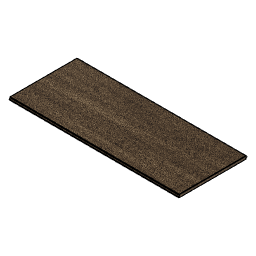
Leaf_Mid (Autodesk Fusion 360 design; units mm, degrees)
Autodesk Fusion 360 part; units mm, degrees
sketch "Sketch1" plane through (0, 0, 0) normal (0, 0, 1) x (1, 0, 0)
  line L0 (-520.7, 210.185) -> (520.7, 210.185)
  line L1 (520.7, 210.185) -> (520.7, -210.185)
  line L2 (520.7, -210.185) -> (-520.7, -210.185)
  line L3 (-520.7, -210.185) -> (-520.7, 210.185)
  line L4 (-520.7, 210.185) -> (520.7, -210.185) construction
  line L5 (520.7, 210.185) -> (-520.7, -210.185) construction
  dimension "d1" = 420.37
  dimension "d2" = 1041.4
  constraint horizontal L0
  constraint perpendicular L0 L1
  constraint parallel L0 L2
  constraint parallel L1 L3
  constraint coincident L4 origin
  constraint coincident L5 origin
  measures "d1" distance of L0.end L1.end
  measures "d2" distance of L0.start L0.end
extrude "Extrude1" add sketch "Sketch1" along normal blind 19.05
sketch "Sketch3" plane through (520.7, 0, 0) normal (1, 0, 0) x (0, 1, 0)
  line L0 (-210.185, 0) -> (210.185, 0)
  line L1 (210.185, 0) -> (210.185, 19.05)
  line L2 (210.185, 19.05) -> (-210.185, 19.05)
  line L3 (-210.185, 19.05) -> (-210.185, 0)
  line L4 (206.375, 0) -> (206.375, 3.175)
  line L5 (206.375, 15.875) -> (206.375, 19.05)
  line L6 (206.375, 3.175) -> (202.565, 4.1959)
  line L7 (202.565, 4.1959) -> (202.565, 8.5041)
  line L8 (202.565, 8.5041) -> (206.375, 9.525)
  line L9 (210.185, 10.5459) -> (210.185, 14.8541) construction
  line L10 (210.185, 14.8541) -> (206.375, 15.875)
  line L11 (206.375, 9.525) -> (210.185, 10.5459)
  line L12 (206.375, 0) -> (210.185, 0)
  line L13 (206.375, 19.05) -> (210.185, 19.05)
  line L14 (210.185, 19.05) -> (210.185, 14.8541)
  line L15 (210.185, 0) -> (210.185, 10.5459)
  line L16 (-202.565, 14.8541) -> (-202.565, 10.5459)
  line L17 (-210.185, 0) -> (-210.185, 4.1959)
  line L18 (-206.375, 19.05) -> (-206.375, 15.875)
  line L19 (-206.375, 9.525) -> (-210.185, 8.5041)
  line L20 (-206.375, 3.175) -> (-206.375, 0)
  line L21 (-206.375, 15.875) -> (-202.565, 14.8541)
  line L22 (-206.375, 19.05) -> (-210.185, 19.05)
  line L23 (-206.375, 0) -> (-210.185, 0)
  line L24 (-210.185, 4.1959) -> (-206.375, 3.175)
  line L25 (-210.185, 19.05) -> (-210.185, 8.5041)
  line L26 (-202.565, 10.5459) -> (-206.375, 9.525)
  line L27 (-210.185, 8.5041) -> (-210.185, 4.1959) construction
  point P0 (210.185, 0)
  dimension "d25" = 105
  dimension "d27" = 19.05
  dimension "d29" = 6.35
  dimension "d30" = 6.35
  dimension "d31" = 3.81
  dimension "d32" = 3.81
  dimension "d33" = 3.81
  dimension "d36" = 105
  dimension "d37" = 19.05
  dimension "d38" = 6.35
  dimension "d39" = 6.35
  dimension "d40" = 3.81
  dimension "d41" = 3.81
  dimension "d42" = 3.81
  constraint vertical L4
  constraint vertical L5
  constraint equal L6 L10
  constraint parallel L6 L10
  constraint equal L4 L5
  constraint equal L7 L9
  constraint equal L8 L11
  constraint equal L6 L8
  constraint perpendicular L9 L12
  constraint perpendicular L5 L13
  constraint perpendicular L13 L14
  constraint perpendicular L12 L15
  constraint equal L21 L24
  constraint parallel L21 L24
  constraint equal L18 L20
  constraint equal L16 L27
  constraint equal L19 L26
  constraint equal L21 L26
  constraint perpendicular L22 L27
  constraint perpendicular L20 L23
  constraint perpendicular L17 L23
  constraint perpendicular L22 L25
  measures "d25" angle of L6 L7
  measures "d27" distance of L4.start L5.end
  measures "d29" distance of L5.start L8.end
  measures "d30" distance of L4.end L8.end
  measures "d31" distance of L7 L8.end
  measures "d32" distance of L9 L8.end
  measures "d33" distance of L4.start P0
  measures "d36" angle of L16 L21
  measures "d37" distance of L20.end L18.start
  measures "d38" distance of L20.start L19.start
  measures "d39" distance of L18.end L19.start
  measures "d40" distance of L19.start L16
  measures "d41" distance of L19.start L27
  measures "d42" distance of L2.end L18.start
extrude "Extrude3" cut sketch "Sketch3" against normal blind 1041.4 contours L0 L3 L17 L20 L23 L24 | L0 L1 L4 L6 L7 L8 L11 L12 L15 | L2 L3 L16 L18 L19 L21 L22 L25 L26 | L1 L2 L5 L10 L13 L14
chamfer "Chamfer1" distance 1.5875 angle 45 8 edges at (-520.7, 0, 19.05) (520.7, 0, 19.05) (-520.7, 0, 0) (520.7, 0, 0) (0, 206.375, 19.05) (0, 206.375, 0) (0, -206.375, 19.05) (0, -206.375, 0)
